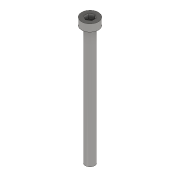
# Autodesk Inventor part: M4_shoulder_bolt
Saved by Autodesk Inventor 2022 (Build 260153000, 153)
## iProperties
Created: 2022-10-12
Part Number: M4_shoulder_bolt
Material: Generic
Document SubType Name: Modeling
Designer: dell
Density: 1 g/cm^3
Appearance: Steel - Polished
Author: dell
Autodesk Inventor part; units mm, degrees
ref_plane "YZ Plane" through (0, 0, 0) normal (1, 0, 0) x (0, 1, 0)
ref_plane "XZ Plane" through (0, 0, 0) normal (0, 1, 0) x (-1, 0, 0)
ref_plane "XY Plane" through (0, 0, 0) normal (0, 0, 1) x (1, 0, 0)
sketch "Sketch1" plane through (0, 0, 0) normal (0, 1, 0) x (-1, 0, 0)
  circle A0 centre (0, 0) radius 2
  dimension "d0" = 4
  constraints: 1 centre point, 1 coincident
  measures "d0" diameter of A0
extrude "Extrusion1" add sketch "Sketch1" along normal blind 50
sketch "Sketch2" plane through (0, 50, 0) normal (0, 1, 0) x (1, 0, 0)
  circle A0 centre (0, 0) radius 3.5
  dimension "d3" = 7
  constraints: 1 centre point, 1 coincident
  measures "d3" diameter of A0
extrude "Extrusion2" add sketch "Sketch2" along normal blind 3
sketch "Sketch3" plane through (0, 53, 0) normal (0, 1, 0) x (1, 0, 0)
  circle A0 centre (0, 0) radius 2 projected
  line L0 (0, 2) -> (1.7321, 1)
  line L1 (1.7321, 1) -> (1.7321, -1)
  line L2 (1.7321, -1) -> (0, -2)
  line L3 (0, -2) -> (-1.7321, -1)
  line L4 (-1.7321, -1) -> (-1.7321, 1)
  line L5 (-1.7321, 1) -> (0, 2)
  constraints: 12 end point, 1 coincident, 1 vertical alignment, 14 other
extrude "Extrusion3" cut sketch "Sketch3" against normal blind 2 contours L1 L2 L3 L4 L5 L0
body "Solid1"
